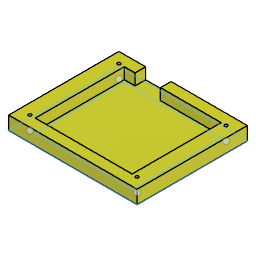
base (Autodesk Fusion 360 design; units mm, degrees)
part number: 2026-02-28-17-25-29-068
Autodesk Fusion 360 part; units mm, degrees
sketch "Sketch4" plane through (0, 0, 0) normal (0, 0, 1) x (1, 0, 0)
  line L0 (-10, 103.05) -> (110, 103.05)
  line L1 (110, 103.05) -> (110, 0)
  line L2 (110, 0) -> (-10, 0)
  line L3 (-10, 0) -> (-10, 103.05)
  line L4 (5, 93.05) -> (95.38, 93.05)
  line L5 (95.38, 93.05) -> (95.38, 10)
  line L6 (95.38, 10) -> (5, 10)
  line L7 (5, 10) -> (5, 93.05)
  circle A0 centre (0, 93.05) radius 1.45
  circle A1 centre (100, 93.05) radius 1.45
  circle A2 centre (100, 10) radius 1.45
  circle A3 centre (0, 10) radius 1.45
  dimension "d9" = 90.38
  dimension "d10" = 83.05
  dimension "d11" = 10
  dimension "d13" = 10
  dimension "d14" = 2.9
  dimension "d15" = 2.9
  dimension "d16" = 2.9
  dimension "d17" = 2.9
  dimension "d50" = 10
  dimension "d51" = 10
  dimension "d52" = 10
  dimension "d53" = 10
  dimension "d54" = 10
  dimension "d55" = 10
  dimension "d56" = 10
  dimension "d57" = 10
  constraint horizontal L0
  constraint vertical L1
  constraint horizontal L2
  constraint vertical L3
  constraint horizontal L4
  constraint vertical L5
  constraint horizontal L6
  constraint vertical L7
  measures "d9" distance of L4.start L4.end
  measures "d10" distance of L4.start L6.end
  measures "d11" vertical distance of L0.end L4.end
  measures "d13" vertical distance of L2.end L6.end
  measures "d14" diameter of A0
  measures "d15" diameter of A1
  measures "d16" diameter of A2
  measures "d17" diameter of A3
  measures "d50" distance of L2 A3.centre
  measures "d51" distance of L3 A3.centre
  measures "d52" distance of L2 A2.centre
  measures "d53" distance of L1 A2.centre
  measures "d54" distance of L1 A1.centre
  measures "d55" distance of L0 A1.centre
  measures "d56" distance of L0 A0.centre
  measures "d57" distance of L3 A0.centre
extrude "Extrude2" add sketch "Sketch4" along normal blind 3
extrude "Extrude3" add 1 faces at (35, 99.7167, 3) along direction (0, 0, 1) blind 10
extrude "Extrude4" add sketch "Sketch4" along normal blind 3 contours L4 L5 L6 L7
move_body "Move4" bodies 1 to x (1, 0, 0) y (0, 1, 0) z (0, 0, 1) at (0, 100, 0)
move_body "Move5" bodies 1 to x (1, 0, 0) y (0, 1, 0) z (0, 0, 1) at (0, -100, 0)
sketch "Sketch8" plane through (0, 103.05, 0) normal (0, 1, 0) x (-1, 0, 0)
  line L0 (-110, 0) -> (10, 0)
  line L1 (10, 0) -> (10, 13)
  line L2 (10, 13) -> (-110, 13)
  line L3 (-110, 13) -> (-110, 0)
  line L4 (-38.6797, 11) -> (-15.0167, 11)
  line L5 (-15.0167, 11) -> (-15.0167, 3)
  line L6 (-15.0167, 3) -> (-38.6797, 3)
  line L7 (-38.6797, 3) -> (-38.6797, 11)
  constraint horizontal L4
  constraint vertical L5
  constraint horizontal L6
  constraint vertical L7
extrude "Extrude8" cut sketch "Sketch8" against normal blind 23 contours L4 L5 L6 L7
move_face "MoveFace1" by (0, 0, -4) 1 faces at (35, 3.3333, 13)
move_face "MoveFace2" by (0, 0, -1) 1 faces at (46.3532, 37.6833, 3)
move_face "MoveFace3" by (0, 0, 4) 1 faces at (35, 3.3333, 9)
move_face "MoveFace4" by (0, 0, -0.5) 1 faces at (35, 3.3333, 13)
named bodies: "bottom case"
